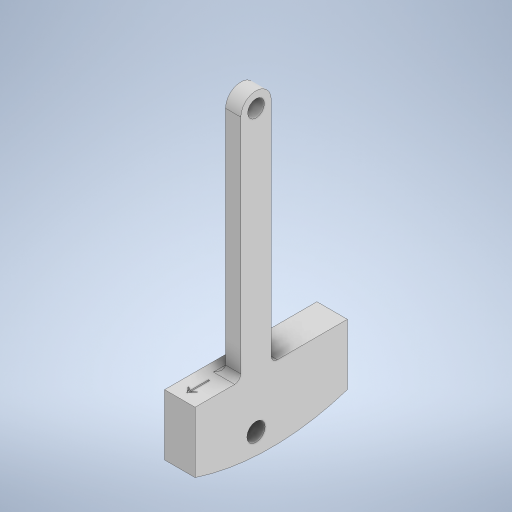
# Autodesk Inventor part: 受動歩行_ver2
Saved by Autodesk Inventor 2023 (Build 270158000, 158)
## iProperties
Created: 2024-05-31
Part Number: 受動歩行_ver2
Material: 一般
Document SubType Name: Modeling
Designer: BABA
Density: 1 g/cm^3
Appearance: 既定
Author: BABA
Autodesk Inventor part; units mm, degrees
ref_plane "YZ Plane" through (0, 0, 0) normal (1, 0, 0) x (0, 1, 0)
ref_plane "XZ Plane" through (0, 0, 0) normal (0, 1, 0) x (-1, 0, 0)
ref_plane "XY Plane" through (0, 0, 0) normal (0, 0, 1) x (1, 0, 0)
sketch "スケッチ1" plane through (0, 0, 0) normal (1, 0, 0) x (0, 1, 0)
  line L0 (-10, 25) -> (10, 25)
  line L1 (10, 25) -> (10, -25)
  line L2 (10, -25) -> (-10, -25)
  line L3 (-10, -25) -> (-10, 25)
  line L4 (-10, 25) -> (10, -25) construction
  line L5 (10, 25) -> (-10, -25) construction
  line L6 (10, 0) -> (-14, 0)
  arc A0 (-10, 25) -> (-10, -25) centre (66.125, 0) ccw
  point P0 (0, 0)
  dimension "d0" = 20
  dimension "d1" = 50
  dimension "d9" = 24
  constraints: 14 end point, 3 midpoint, 3 point on circle, 2 parallel, 2 perpendicular, 1 centre point, 1 horizontal
  measures "d0" distance of L1.end L2.end
  measures "d1" distance of L0.end L1.end
  measures "d9" distance of L6.start L6.end
extrude "押し出し1" add sketch "スケッチ1" against normal blind 10
sketch "スケッチ2" plane through (0, 0, 0) normal (1, 0, 0) x (0, 0, -1)
  line L0 (-25, 10) -> (25, 10) projected
  line L1 (-10, 10) -> (0, 10)
  line L2 (0, 10) -> (0, 90)
  line L3 (0, 90) -> (-10, 90)
  line L4 (-10, 90) -> (-10, 10)
  point P0 (0, 0)
  point P1 (0, 10)
  dimension "d4" = 10
  dimension "d5" = 80
  dimension "d6" = 10
  constraints: 8 end point, 2 parallel, 1 horizontal, 1 perpendicular, 1 point on line
  measures "d4" distance of L3.end L2.end
  measures "d5" distance of L2.end L1.end
  measures "d6" distance from line of L4 point (0, 0)
extrude "押し出し2" add sketch "スケッチ2" against normal blind 5
sketch "スケッチ3" plane through (0, 0, 0) normal (1, 0, 0) x (0, 0, -1)
  line L0 (25, 10) -> (0, 10) projected
  point P0 (0, 0)
  point P1 (-5, -7)
  dimension "d12" = 5
  dimension "d13" = 7
  measures "d12" horizontal distance of point (-5, -7) point (0, 0)
  measures "d13" vertical distance of point (0, 0) point (-5, -7)
hole "穴1" at (0, -7, 5) direction (-1, 0, 0) diameter 6 end through all
sketch "スケッチ4" plane through (0, 0, 0) normal (1, 0, 0) x (0, 0, -1)
  line L0 (0, 90) -> (-10, 90) projected
  line L1 (0, 10) -> (0, 90) projected
  point P0 (0, 0)
  point P1 (-5, 85)
  point P2 (-5, 90)
  dimension "d21" = 5
  dimension "d22" = 5
  constraints: 1 midpoint
  measures "d21" distance of point (-5, 90) point (-5, 85)
  measures "d22" distance from line of L1 point (-5, 85)
hole "穴2" at (0, 85, 5) direction (-1, 0, 0) diameter 5.5 end through all
fillet "フィレット1" radius 2 3 edges at (-2.5, 10, 0) (-5, 10, 5) (-2.5, 10, 10)
fillet "フィレット2" radius 5 2 edges at (-2.5, 90, 0) (-2.5, 90, 10)
sketch "スケッチ5" plane through (-10, 10, -25) normal (0, 1, 0) x (1, 0, 0)
  line L0 (2.5, -40) -> (7.5, -40) construction
  line L1 (7.5, -40) -> (7.5, -45) construction
  line L2 (7.5, -45) -> (2.5, -45) construction
  line L3 (2.5, -45) -> (2.5, -40) construction
  line L4 (10, -37) -> (10, -50) projected
  line L5 (10, -50) -> (0, -50) projected
  line L6 (3.1278, -45.5513) -> (3.1278, -45.2399)
  spline S0 degree 2 poles (3.1278, -45.2399) (3.6122, -45.4821) (3.9978, -45.7293) (4.3933, -46.0407) knots 0 0 0 1 2 2 2
  line L7 (4.3933, -46.0407) -> (4.3933, -40)
  line L8 (4.3933, -40) -> (4.8085, -40)
  line L9 (4.8085, -40) -> (4.8085, -46.0407)
  spline S1 degree 2 poles (4.8085, -46.0407) (5.2485, -45.6156) (6.074, -45.23) knots 0 0 0 1 1 1
  line L10 (6.074, -45.23) -> (6.074, -45.5464)
  spline S2 degree 2 poles (6.074, -45.5464) (5.4808, -46.0753) (4.8728, -46.8365) (4.68, -47.2419) knots 0 0 0 1 2 2 2
  line L11 (4.68, -47.2419) -> (4.4921, -47.2419)
  spline S3 degree 2 poles (4.4921, -47.2419) (4.3389, -46.8909) (3.721, -46.0951) (3.1278, -45.5513) knots 0 0 0 1 2 2 2
  point P0 (10, -25)
  point P1 (7.5, -42.5)
  dimension "d34" = 2.5
  dimension "d35" = 5
  dimension "d36" = 5
  dimension "d37" = 5
  constraints: 1 midpoint, 2 other
  measures "d34" distance from line of L4 point (7.5, -42.5)
  measures "d35" distance between parallel lines of L5 L2
  measures "d36" distance of L1.end L2.end
  measures "d37" distance of L2.end L0.start
extrude "押し出し3" cut sketch "スケッチ5" against normal blind 1
